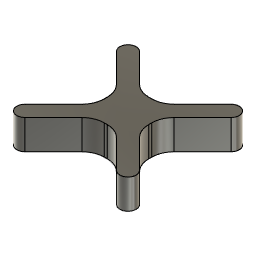
Grip Screw Head v8 (Autodesk Fusion 360 design; units mm, degrees)
Autodesk Fusion 360 part; units mm, degrees
sketch "Sketch1" plane through (0, 0, 0) normal (0, 0, 1) x (1, 0, 0)
  line L0 (9.6, 5.5426) -> (0, 11.0851)
  line L1 (0, 11.0851) -> (-9.6, 5.5426)
  line L2 (-9.6, 5.5426) -> (-9.6, -5.5426)
  line L3 (-9.6, -5.5426) -> (0, -11.0851)
  line L4 (0, -11.0851) -> (9.6, -5.5426)
  line L5 (9.6, -5.5426) -> (9.6, 5.5426)
  line L6 (-15, 15) -> (15, 15)
  line L7 (15, 15) -> (15, -15)
  line L8 (15, -15) -> (-15, -15)
  line L9 (-15, -15) -> (-15, 15)
  line L10 (-6.1109, 13.8891) -> (-30.8597, 38.6378)
  arc A0 (-30.8597, 38.6378) -> (-38.6378, 30.8597) centre (-34.7487, 34.7487) ccw
  line L11 (-38.6378, 30.8597) -> (-13.8891, 6.1109)
  arc A1 (-13.8891, 6.1109) -> (-6.1109, 13.8891) centre (-10, 10) ccw
  line L12 (-10, 10) -> (-34.7487, 34.7487) construction
  line L13 (13.8891, 6.1109) -> (38.6378, 30.8597)
  arc A2 (38.6378, 30.8597) -> (30.8597, 38.6378) centre (34.7487, 34.7487) ccw
  line L14 (30.8597, 38.6378) -> (6.1109, 13.8891)
  arc A3 (6.1109, 13.8891) -> (13.8891, 6.1109) centre (10, 10) ccw
  line L15 (10, 10) -> (34.7487, 34.7487) construction
  line L16 (-13.8891, -6.1109) -> (-38.6378, -30.8597)
  arc A4 (-38.6378, -30.8597) -> (-30.8597, -38.6378) centre (-34.7487, -34.7487) ccw
  line L17 (-30.8597, -38.6378) -> (-6.1109, -13.8891)
  arc A5 (-6.1109, -13.8891) -> (-13.8891, -6.1109) centre (-10, -10) ccw
  line L18 (-10, -10) -> (-34.7487, -34.7487) construction
  line L19 (6.1109, -13.8891) -> (30.8597, -38.6378)
  arc A6 (30.8597, -38.6378) -> (38.6378, -30.8597) centre (34.7487, -34.7487) ccw
  line L20 (38.6378, -30.8597) -> (13.8891, -6.1109)
  arc A7 (13.8891, -6.1109) -> (6.1109, -13.8891) centre (10, -10) ccw
  line L21 (10, -10) -> (34.7487, -34.7487) construction
  dimension "d1" = 9.6
  dimension "d2" = 11
  dimension "d3" = 11
  dimension "d4" = 11
  dimension "d5" = 35
  dimension "d7" = 11
  dimension "d10" = 35
  dimension "d11" = 35
  dimension "d12" = 35
  constraint horizontal L6
  constraint vertical L7
  constraint horizontal L8
  constraint vertical L9
  constraint tangent L10 A0
  constraint tangent A0 L11
  constraint parallel L10 L11
  constraint tangent L11 A1
  constraint tangent L10 A1
  constraint tangent L13 A2
  constraint tangent A2 L14
  constraint parallel L13 L14
  constraint tangent L14 A3
  constraint tangent L13 A3
  constraint tangent L16 A4
  constraint tangent A4 L17
  constraint parallel L16 L17
  constraint tangent L17 A5
  constraint tangent L16 A5
  constraint tangent L19 A6
  constraint tangent A6 L20
  constraint parallel L19 L20
  constraint tangent L20 A7
  constraint tangent L19 A7
  measures "d1" distance of origin L5
  measures "d2" diameter of A0
  measures "d3" diameter of A2
  measures "d4" diameter of A4
  measures "d5" distance of A7.centre A6.centre
  measures "d7" diameter of A6
  measures "d10" distance of A3.centre A2.centre
  measures "d11" distance of A5.centre A4.centre
  measures "d12" distance of A1.centre A0.centre
extrude "Extrude1" add sketch "Sketch1" along normal blind 20 contours L0 L5 L6 L7 L13 L14 A3 | L0 L1 L6 L10 A1 L14 A3 | L5 L7 L13 A3 L20 A7 | L4 L5 L7 L8 L19 L20 A7 | L1 L2 L6 L9 L10 L11 A1 | L6 L7 L13 A2 L14 | L3 L4 L8 L17 A5 L19 A7 | L2 L9 L11 A1 L16 A5 | L6 L9 L10 A0 L11 | L7 L8 L19 A6 L20 | L2 L3 L8 L9 L16 L17 A5 | L8 L9 L16 A4 L17
sketch "Sketch2" plane through (0, 0, 20) normal (0, 0, 1) x (-1, 0, 0)
  line L0 (-9.6, -5.5426) -> (-9.6, 5.5426)
  line L1 (-9.6, 5.5426) -> (0, 11.0851)
  line L2 (0, 11.0851) -> (9.6, 5.5426)
  line L3 (9.6, 5.5426) -> (9.6, -5.5426)
  line L4 (9.6, -5.5426) -> (0, -11.0851)
  line L5 (0, -11.0851) -> (-9.6, -5.5426)
  line L6 (-7.2218, 15) -> (-30.8597, 38.6378)
  arc A0 (-30.8597, 38.6378) -> (-38.6378, 30.8597) centre (-34.7487, 34.7487) ccw
  line L7 (-38.6378, 30.8597) -> (-15, 7.2218)
  line L8 (-15, 7.2218) -> (-15, -7.2218)
  line L9 (-15, -7.2218) -> (-38.6378, -30.8597)
  arc A1 (-38.6378, -30.8597) -> (-30.8597, -38.6378) centre (-34.7487, -34.7487) ccw
  line L10 (-30.8597, -38.6378) -> (-7.2218, -15)
  line L11 (-7.2218, -15) -> (7.2218, -15)
  line L12 (7.2218, -15) -> (30.8597, -38.6378)
  arc A2 (30.8597, -38.6378) -> (38.6378, -30.8597) centre (34.7487, -34.7487) ccw
  line L13 (38.6378, -30.8597) -> (15, -7.2218)
  line L14 (15, -7.2218) -> (15, 7.2218)
  line L15 (15, 7.2218) -> (38.6378, 30.8597)
  arc A3 (38.6378, 30.8597) -> (30.8597, 38.6378) centre (34.7487, 34.7487) ccw
  line L16 (30.8597, 38.6378) -> (7.2218, 15)
  line L17 (7.2218, 15) -> (-7.2218, 15)
extrude "Extrude2" add sketch "Sketch2" against normal blind 12 contours L0 L1 L2 L3 L4 L5
fillet "Fillet1" radius 15 8 edges at (-7.2218, 15, 10) (7.2218, 15, 10) (15, 7.2218, 10) (15, -7.2218, 10) (7.2218, -15, 10) (-7.2218, -15, 10) (-15, -7.2218, 10) (-15, 7.2218, 10)
equation "d1 = ( 19.2 / 2 ) * 1 mm"
